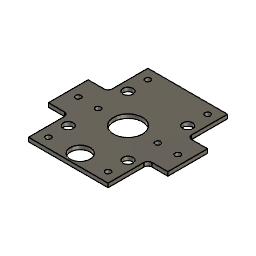
receiver_support_txclose (Autodesk Fusion 360 design; units mm, degrees)
Autodesk Fusion 360 part; units mm, degrees
sketch "Sketch1" plane through (0, 0, 0) normal (0, 0, 1) x (1, 0, 0)
  line L0 (0, 0) -> (40, 0)
  line L1 (40, 0) -> (40, 60)
  line L2 (40, 60) -> (0, 60)
  line L3 (0, 60) -> (0, 0)
  circle A0 centre (5, 5) radius 1.35
  circle A1 centre (20, 30) radius 7.25
  circle A2 centre (20, 30) radius 5.75
  circle A3 centre (35, 5) radius 1.35
  circle A4 centre (5, 30) radius 1.35
  circle A5 centre (35, 30) radius 1.35
  circle A6 centre (5, 55) radius 1.35
  circle A7 centre (35, 55) radius 1.35
  circle A8 centre (20, 6) radius 5
  line L4 (-10, 40) -> (50, 40)
  line L5 (50, 40) -> (50, 20)
  line L6 (50, 20) -> (-10, 20)
  line L7 (-10, 20) -> (-10, 40)
  circle A9 centre (-5, 30) radius 1.35
  circle A10 centre (45, 30) radius 1.35
  dimension "d1" = 2.7
  dimension "d2" = 60
  dimension "d3" = 40
  dimension "d4" = 5
  dimension "d5" = 5
  dimension "d6" = 14.5
  dimension "d7" = 20
  dimension "d8" = 30
  dimension "d9" = 11.5
  dimension "d12" = 30
  dimension "d13" = 50
  dimension "d20" = 6
  dimension "d21" = 20
  dimension "d22" = 10
  dimension "d23" = 60
  dimension "d24" = 20
  dimension "d25" = 30
  dimension "d26" = 10
  dimension "d29" = 50
  dimension "d30" = 0
  dimension "d31" = 2.7
  dimension "d32" = 5
  dimension "d33" = 10
  constraint horizontal L0
  constraint vertical L1
  constraint horizontal L2
  constraint vertical L3
  constraint coincident L0.start L3.end
  constraint concentric A1 A2
  constraint horizontal L4
  constraint vertical L5
  constraint horizontal L6
  constraint vertical L7
  measures "d1" diameter of A0
  measures "d2" distance of L0.end L1.end
  measures "d3" distance of L1.end L2.end
  measures "d4" distance of L0 A0.centre
  measures "d5" distance of L3 A0.centre
  measures "d6" diameter of A1
  measures "d7" distance of L1 A1.centre
  measures "d8" distance of L0 A1.centre
  measures "d9" diameter of A2
  measures "d20" distance of L0 A8.centre
  measures "d21" distance of L1 A8.centre
  measures "d22" diameter of A8
  measures "d23" distance of L4.start L4.end
  measures "d24" distance of L4.start L6.end
  measures "d25" distance of A1.centre L7
  measures "d26" distance of A1.centre L4
  measures "d31" diameter of A9
  measures "d32" distance of L7 A9.centre
  measures "d33" distance of L4 A9.centre
extrude "Extrude1" add sketch "Sketch1" along normal blind 2 contours L0 L1 L3 L6 | L3 L4 L6 L7 | L1 L3 L4 L6 | L1 L4 L5 L6 | L1 L2 L3 L4
fillet "Fillet2" radius 2 4 edges at (40, 20, 1) (40, 40, 1) (0, 40, 1) (0, 20, 1)
sketch "Sketch2" plane through (0, 0, 2) normal (0, 0, 1) x (-1, 0, 0)
  circle A0 centre (-5, -5) radius 1.35
  circle A1 centre (-5, -30) radius 1.35
  circle A2 centre (-35, -5) radius 1.35
  circle A3 centre (-35, -30) radius 1.35
  circle A4 centre (-35, -55) radius 1.35
  circle A5 centre (-20, -6) radius 5
  circle A6 centre (-20, -30) radius 7.25
  circle A7 centre (-45, -30) radius 1.35
  circle A8 centre (5, -30) radius 1.35
  circle A9 centre (-5, -55) radius 1.35
  line L0 (0, -18) -> (0, 0)
  line L1 (0, 0) -> (-40, 0)
  line L2 (-40, 0) -> (-40, -18)
  arc A10 (-42, -20) -> (-40, -18) centre (-42, -18) ccw
  line L3 (-42, -20) -> (-50, -20)
  line L4 (-50, -20) -> (-50, -40)
  line L5 (-50, -40) -> (-42, -40)
  arc A11 (-40, -42) -> (-42, -40) centre (-42, -42) ccw
  line L6 (-40, -42) -> (-40, -60)
  line L7 (-40, -60) -> (0, -60)
  line L8 (0, -60) -> (0, -42)
  arc A12 (2, -40) -> (0, -42) centre (2, -42) ccw
  line L9 (2, -40) -> (10, -40)
  line L10 (10, -40) -> (10, -20)
  line L11 (10, -20) -> (2, -20)
  arc A13 (0, -18) -> (2, -20) centre (2, -18) ccw
  circle A14 centre (-5, -45) radius 2.5
  circle A15 centre (-35, -45) radius 2.5
  circle A16 centre (-5, -15) radius 2.5
  circle A17 centre (-35, -15) radius 2.5
  dimension "d38" = -30
  dimension "d39" = 30
  dimension "d40" = 5
  dimension "d41" = 15
  dimension "d42" = 5
  measures "d40" diameter of A14
  measures "d41" distance of A1.centre A14.centre
  measures "d42" distance of L8 A14.centre
extrude "Extrude3" cut sketch "Sketch2" against normal blind 2 contours A14 | A15 | A16 | A17
extrude "Extrude2" [suppressed]
fillet "Fillet1" [suppressed]
